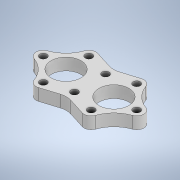
# Autodesk Inventor part: Part6
Saved by Autodesk Inventor 2021 (Build 250183000, 183)
## iProperties
Created: 2022-04-24
Part Number: Part6
Material: Generic
Document SubType Name: Modeling
Designer: hp
Density: 1 g/cm^3
Appearance: Default
Author: hp
Autodesk Inventor part; units mm, degrees
ref_plane "YZ Plane" through (0, 0, 0) normal (1, 0, 0) x (0, 1, 0)
ref_plane "XZ Plane" through (0, 0, 0) normal (0, 1, 0) x (-1, 0, 0)
ref_plane "XY Plane" through (0, 0, 0) normal (0, 0, 1) x (1, 0, 0)
sketch "Sketch1" plane through (0, 0, 0) normal (0, 1, 0) x (-1, 0, 0)
  circle A0 centre (0, 0) radius 12.5
  arc A1 (20.9848, -5.6622) -> (20.9848, 5.6622) centre (19, 0) ccw
  arc A2 (5.6622, 20.9848) -> (-5.9247, 18.0526) centre (0, 19) ccw
  arc A3 (-5.9247, -18.0526) -> (5.6622, -20.9848) centre (0, -19) ccw
  arc A4 (5.6622, 20.9848) -> (20.9848, 5.6622) centre (29.2547, 29.2547) ccw
  arc A5 (20.9848, -5.6622) -> (5.6622, -20.9848) centre (29.2547, -29.2547) ccw
  line L0 (-20, 15) -> (-20, -19.7218)
  line L1 (-20, 15) -> (-20, 19.7218)
  circle A6 centre (-20, 13) radius 3
  circle A7 centre (-20, -13) radius 3
  line L2 (-20, 0) -> (-15, 0)
  circle A8 centre (0, 19) radius 3
  circle A9 centre (19, 0) radius 3
  circle A10 centre (0, -19) radius 3
  circle A11 centre (-40, 0) radius 12.5
  arc A12 (-60.9848, 5.6622) -> (-60.9848, -5.6622) centre (-59, 0) ccw
  arc A13 (-37.8834, 24.6143) -> (-45.6622, 20.9848) centre (-40, 19) ccw
  arc A14 (-45.6622, -20.9848) -> (-37.8834, -24.6143) centre (-40, -19) ccw
  arc A15 (-60.9848, 5.6622) -> (-45.6622, 20.9848) centre (-69.2547, 29.2547) ccw
  arc A16 (-45.6622, -20.9848) -> (-60.9848, -5.6622) centre (-69.2547, -29.2547) ccw
  circle A17 centre (-20, 13) radius 3
  circle A18 centre (-20, -13) radius 3
  line L3 (-20, 0) -> (-25, 0)
  circle A19 centre (-40, 19) radius 3
  circle A20 centre (-59, 0) radius 3
  circle A21 centre (-40, -19) radius 3
  line L4 (-15.5071, 20.4105) -> (-1.4719, 24.8166)
  line L5 (-24.4929, 20.4105) -> (-38.5281, 24.8166)
  line L6 (-1.4719, -24.8166) -> (-15.5071, -20.4105)
  line L7 (-38.5281, -24.8166) -> (-24.4929, -20.4105)
  arc A22 (-20.599, 19.1881) -> (-19.401, 19.1881) centre (-20, 21.0962) ccw
  arc A23 (-24.4929, 20.4105) -> (-15.5071, 20.4105) centre (-20, 34.7218) ccw
  arc A24 (-15.5071, -20.4105) -> (-24.4929, -20.4105) centre (-20, -34.7218) ccw
  point P0 (-34.0753, 18.0526)
  point P1 (-34.0753, -18.0526)
  point P2 (-20, 19)
  point P3 (-20, -19)
  dimension "d46" = 25
  dimension "d48" = 12
  dimension "d49" = 12
  dimension "d50" = 12
  dimension "d51" = 50
  dimension "d52" = 26.8701
  dimension "d53" = 26.8701
  dimension "d54" = 50
  dimension "d55" = 20
  dimension "d56" = 6
  dimension "d57" = 6
  dimension "d58" = 13
  dimension "d59" = 13
  dimension "d60" = 6
  dimension "d61" = 6
  dimension "d62" = 6
  dimension "d65" = 19
  dimension "d66" = 19
  dimension "d67" = 19
  dimension "d68" = 6
  dimension "d69" = 6
  dimension "d70" = 2
  dimension "d71" = 15
  constraints: 32 point on circle, 25 centre point, 16 end point, 16 symmetric about line, 13 point on line, 10 tangent, 4 coincident, 2 parallel, 2 vertical, 1 concentric, 1 equal radius, 1 horizontal, 11 other
  measures "d46" diameter of A0
  measures "d48" diameter of A1
  measures "d49" diameter of A3
  measures "d50" diameter of A2
  measures "d51" diameter of A4
  measures "d52" distance of A1.centre A2.centre
  measures "d53" distance of A3.centre A1.centre
  measures "d54" diameter of A5
  measures "d55" distance from line of L0 A0.centre
  measures "d56" diameter of A7
  measures "d57" diameter of A6
  measures "d58" distance of L2.start A6.centre
  measures "d59" distance of A7.centre L2.start
  measures "d60" diameter of A9
  measures "d61" diameter of A8
  measures "d62" diameter of A10
  measures "d65" distance of A0.centre A1.centre
  measures "d66" distance of A0.centre A2.centre
  measures "d67" distance of A3.centre A0.centre
  measures "d68" distance of A6.centre point (-20, 19)
  measures "d69" distance of A7.centre point (-20, -19)
  measures "d70" radius of A22
  measures "d71" radius of A23
extrude "Extrusion1" add sketch "Sketch1" along normal blind 10 contours A5 A3 L6 A24 L0 A7 A6 L1 A23 L4 A2 A4 A1 | A24 L7 A14 A16 A12 A15 A13 L5 A23 L1 A6 L0 A7
equation "\"d49\" = d48"
equation "\"d50\" = d48"
equation "\"d59\" = d58"
equation "\"d28\" = d27"
equation "\"d29\" = d28"
equation "\"d30\" = d29"
equation "\"d27\" = 72deg"
body "Solid1"
